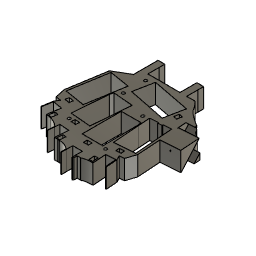
Copy_v4 (Autodesk Fusion 360 design; units mm, degrees)
Autodesk Fusion 360 part; units mm, degrees
note: some values were not read from the file. Set by a fixed rule: which sketch regions a step uses.
other "Base Mesh Feature1"
sketch "Sketch1" plane through (0, 0, 0.01) normal (0, 0, 1) x (1, 0, 0)
  line L0 (36.0813, -1.8889) -> (32.9752, 43.2487)
  line L1 (32.7513, -12.1179) -> (36.0813, -1.8889)
  line L2 (27.6845, -12.4899) -> (32.7513, -12.1179)
  line L3 (30.0654, -16.8996) -> (27.6845, -12.4899)
  line L4 (30.9849, -29.0009) -> (30.0654, -16.8996)
  line L5 (29.4427, -17.4772) -> (30.3023, -29.0109)
  line L6 (19.6436, -18.2077) -> (29.4427, -17.4772)
  line L7 (20.6901, -32.2445) -> (19.6436, -18.2077)
  line L8 (6.3028, -33.911) -> (9.753, -33.9098)
  line L9 (6.3027, -37.2346) -> (6.3028, -33.911)
  line L10 (5.577, -37.9174) -> (6.3027, -37.2346)
  line L11 (4.9263, -37.9059) -> (5.577, -37.9174)
  line L12 (4.9132, -27.2369) -> (4.9059, -37.8615)
  line L13 (-4.9131, -27.2369) -> (4.9132, -27.2369)
  line L14 (-4.9303, -38.8327) -> (-4.9131, -27.2369)
  line L15 (-5.5394, -38.808) -> (-4.9303, -38.8327)
  line L16 (-5.5099, -33.2116) -> (-5.5394, -38.808)
  line L17 (-18.1322, -29.3561) -> (-16.5345, -29.3675)
  line L18 (-21.6433, -29.2745) -> (-18.1322, -29.3561)
  line L19 (-20.4904, -15.7696) -> (-21.6433, -29.2745)
  line L20 (-30.2811, -14.9338) -> (-20.4904, -15.7696)
  line L21 (-31.2834, -26.4889) -> (-30.2811, -14.9338)
  line L22 (-31.7337, -26.4423) -> (-31.2834, -26.4889)
  line L23 (-31.1662, -19.694) -> (-31.7337, -26.4423)
  line L24 (-46.0317, -13.0034) -> (-45.6993, -13.1615)
  line L25 (-43.8507, 0.1867) -> (-46.0317, -13.0034)
  line L26 (-53.5454, 1.7898) -> (-43.8507, 0.1867)
  line L27 (-55.2865, -8.7399) -> (-53.5454, 1.7898)
  line L28 (-55.8526, -8.6917) -> (-55.2865, -8.7399)
  line L29 (-54.0371, 2.3883) -> (-55.8526, -8.6917)
  line L30 (-51.2811, 6.5583) -> (-54.0371, 2.3883)
  line L31 (-56.4897, 7.4399) -> (-51.2811, 6.5583)
  line L32 (-58.7948, 17.9104) -> (-56.4897, 7.4399)
  line L33 (-52.3403, 57.6045) -> (-58.7948, 17.9104)
  line L34 (-36.826, 66.678) -> (-52.3403, 57.6045)
  line L35 (-36.8289, 85.8904) -> (-36.826, 66.678)
  line L36 (-29.9469, 74.4662) -> (-29.9469, 85.8904)
  line L37 (2.7431, 74.4567) -> (-29.9469, 74.4662)
  line L38 (2.7431, 85.8904) -> (2.7431, 74.4567)
  line L39 (9.6191, 85.8904) -> (2.7431, 85.8904)
  line L40 (9.6191, 74.4567) -> (9.6191, 85.8904)
  line L41 (18.0806, 74.4608) -> (9.6191, 74.4567)
  line L42 (40.9354, 52.3159) -> (40.995, 53.4081)
  line L43 (43.4569, 50.4105) -> (40.9354, 52.3159)
  line L44 (44.0171, 50.8716) -> (43.4569, 50.4105)
  line L45 (42.0183, 41.437) -> (45.9172, 41.6472)
  line L46 (32.9752, 43.2487) -> (42.0183, 41.437)
  line L47 (20.5159, 63.3141) -> (16.3615, 42.6858)
  line L48 (-18.6487, 70.9533) -> (20.5159, 63.3141)
  line L49 (-22.6664, 50.5546) -> (-18.6487, 70.9533)
  line L50 (16.3615, 42.6858) -> (-22.6664, 50.5546)
  line L51 (4.9059, -37.8615) -> (4.9263, -37.9059)
  spline S0 degree 5 poles (45.9172, 41.6472) (46.0239, 42.1861) (46.222, 43.1941) (46.4734, 44.4972) (46.6984, 45.8908) (46.6354, 47.3689) (46.0898, 48.5946) (45.2491, 49.6596) (44.4651, 50.4535) (44.0171, 50.8716) knots 0 0 0 0 0 0 0.2 0.4 0.6 0.8 1 1 1 1 1 1
  line L52 (45.063, 49.8956) -> (42.9712, 51.8475)
  line L53 (45.6555, 40.3248) -> (46.179, 42.9695)
  line L54 (-29.9469, 85.8904) -> (-36.8289, 85.8904)
  line L55 (9.7581, -34.0874) -> (9.753, -33.9098)
  line L56 (30.9849, -29.0009) -> (30.3023, -29.0109)
  spline S1 degree 5 poles (40.995, 53.4081) (38.5459, 54.9422) (34.2281, 57.7327) (29.4904, 61.0866) (26.0623, 64.1864) (24.207, 66.9799) (22.775, 69.3323) (20.8665, 71.6268) (19.0929, 73.4647) (18.0806, 74.4608) knots 0 0 0 0 0 0 0.2 0.4 0.6 0.8 1 1 1 1 1 1
  line L57 (47.1881, 49.5288) -> (34.8019, 57.2874)
  line L58 (20.6612, 71.9215) -> (15.5, 77)
  spline S2 degree 5 poles (20.6901, -32.2445) (20.1069, -32.2354) (18.9879, -32.2293) (17.4506, -32.2564) (15.6408, -32.3648) (13.618, -32.6511) (12.0778, -33.0579) (10.9226, -33.5077) (10.1472, -33.8818) (9.7581, -34.0874) knots 0 0 0 0 0 0 0.2 0.4 0.6 0.8 1 1 1 1 1 1
  line L59 (10.7258, -33.576) -> (8.7904, -34.5988)
  line L60 (22.1647, -32.2674) -> (19.2154, -32.2215)
  line L61 (18.766, -24.9684) -> (19.1881, -30.9501)
  line L62 (15.1693, -25.251) -> (18.766, -24.9684)
  line L63 (15.5913, -31.2369) -> (15.1693, -25.251)
  line L64 (19.1881, -30.9501) -> (15.5913, -31.2369)
  line L65 (-2.4635, -18.739) -> (2.4519, -18.7391)
  line L66 (-2.4564, -14.9483) -> (-2.4635, -18.739)
  line L67 (2.4519, -14.9483) -> (-2.4564, -14.9483)
  line L68 (2.4519, -18.7391) -> (2.4519, -14.9483)
  line L69 (21.4548, -9.5512) -> (26.3566, -9.1859)
  line L70 (21.1801, -5.7705) -> (21.4548, -9.5512)
  line L71 (26.0748, -5.4057) -> (21.1801, -5.7705)
  line L72 (26.3566, -9.1859) -> (26.0748, -5.4057)
  line L73 (-16.2753, -22.8856) -> (-16.7887, -28.8562)
  line L74 (-19.6716, -22.5382) -> (-16.2753, -22.8856)
  line L75 (-20.1856, -28.5134) -> (-19.6716, -22.5382)
  line L76 (-16.7887, -28.8562) -> (-20.1856, -28.5134)
  line L77 (-21.8975, -3.3162) -> (-22.2199, -7.0932)
  line L78 (-26.7951, -2.8981) -> (-21.8975, -3.3162)
  line L79 (-27.1175, -6.6751) -> (-26.7951, -2.8981)
  line L80 (-22.2199, -7.0932) -> (-27.1175, -6.6751)
  spline S3 degree 5 poles (-5.5099, -33.2116) (-5.8497, -32.9739) (-6.5527, -32.5017) (-7.6769, -31.8034) (-9.3011, -30.9072) (-11.507, -29.9489) (-13.4115, -29.4433) (-14.9328, -29.2986) (-15.993, -29.3242) (-16.5345, -29.3675) knots 0 0 0 0 0 0 0.2 0.4 0.6 0.8 1 1 1 1 1 1
  line L81 (-4.6593, -33.8068) -> (-6.3605, -32.6165)
  line L82 (-15.2099, -29.2615) -> (-17.8592, -29.4735)
  spline S4 degree 5 poles (-31.1662, -19.694) (-31.3545, -19.3593) (-31.8362, -18.6888) (-32.8739, -17.6793) (-34.8089, -16.3455) (-37.895, -14.8239) (-40.7733, -13.8723) (-43.148, -13.4044) (-44.832, -13.2211) (-45.6993, -13.1615) knots 0 0 0 0 0 0 0.2 0.4 0.6 0.8 1 1 1 1 1 1
  line L83 (-43.5543, -13.3088) -> (-47.8443, -13.0143)
  line L84 (-30.7289, -20.4713) -> (-31.6035, -18.9166)
  line L85 (-40.0467, -7.1995) -> (-41.0386, -13.1166)
  line L86 (-43.5618, -6.6259) -> (-40.0467, -7.1995)
  line L87 (-44.5531, -12.5388) -> (-43.5618, -6.6259)
  line L88 (-41.0386, -13.1166) -> (-44.5531, -12.5388)
  circle A0 centre (-30.7678, -4.9879) radius 1.4659
  circle A1 centre (14.7861, -13.3473) radius 1.4659
  line L89 (-10.5247, -12.0229) -> (10.5003, -12.0259)
  line L90 (-10.5102, 27.8914) -> (-10.5247, -12.0229)
  line L91 (9.6517, 27.8914) -> (-10.5102, 27.8914)
  line L92 (10.1905, 24.0869) -> (9.6517, 27.8914)
  line L93 (10.5003, -12.0259) -> (10.1905, 24.0869)
  line L94 (22.4476, 37.2561) -> (30.9201, 37.9127)
  line L95 (30.9201, 37.9127) -> (33.9307, -1.9021)
  line L96 (33.9307, -1.9021) -> (12.9473, -3.4609)
  line L97 (12.9473, -3.4609) -> (9.9887, 36.3068)
  line L98 (9.9887, 36.3068) -> (18.4543, 36.9595)
  line L99 (18.4543, 36.9595) -> (18.5275, 35.9515)
  line L100 (18.5275, 35.9515) -> (22.5161, 36.2534)
  line L101 (22.5161, 36.2534) -> (22.4476, 37.2561)
  line L102 (-10.2152, 38.6652) -> (-13.611, -1.0998)
  line L103 (-30.4568, 40.4222) -> (-10.2152, 38.6652)
  line L104 (-31.4926, 36.7486) -> (-30.4568, 40.4222)
  line L105 (-34.5584, 0.7056) -> (-31.4926, 36.7486)
  line L106 (-13.611, -1.0998) -> (-34.5584, 0.7056)
  circle A2 centre (4.6568, 34.6748) radius 1.5
  line L107 (-44.8927, 8.9723) -> (-49.7422, 9.7741)
  line L108 (-49.7422, 9.7741) -> (-49.1168, 13.5129)
  line L109 (-49.1168, 13.5129) -> (-44.2743, 12.7122)
  line L110 (-44.2743, 12.7122) -> (-44.8927, 8.9723)
  line L111 (-35.8494, 14.2954) -> (-56.6063, 17.7506)
  line L112 (-56.6063, 17.7506) -> (-50.1165, 56.9742)
  line L113 (-50.1165, 56.9742) -> (-29.3405, 53.5561)
  line L114 (-29.3405, 53.5561) -> (-35.8494, 14.2954)
  line L115 (24.536, 49.2635) -> (20.8213, 50.0184)
  line L116 (20.8213, 50.0184) -> (21.7896, 54.8302)
  line L117 (21.7896, 54.8302) -> (25.5057, 54.0823)
  line L118 (25.5057, 54.0823) -> (24.536, 49.2635)
  circle A3 centre (-25.4932, 45.1036) radius 1.5
  circle A4 centre (-25.2593, 67.4913) radius 1.5
  constraint midpoint L44.start L52
  constraint midpoint L45.end L53
  constraint midpoint L42.end L57
  constraint midpoint L41.start L58
  constraint midpoint L55.start L59
  constraint midpoint L7.start L60
  constraint midpoint L16.start L81
  constraint midpoint L17.end L82
  constraint midpoint L24.end L83
  constraint midpoint L23.start L84
other "MeshSection1"
extrude "Extrude1" add sketch "Sketch1" along normal blind 19.73 makes body 1
extrude "Extrude2" add 1 faces at (7.3271, 85.8904, 6.5867) along direction (-0.000001, 1, 0) blind 5.8 on bodies 1 bodies 1
extrude "Extrude3" add 1 faces at (-34.5349, 85.8904, 13.1633) along direction (-0.000001, 1, 0) blind 5.8 on bodies 1 bodies 1
other "GenerateFaceGroups1"
sketch "Sketch1 (2)" plane through (0, 0, 0.01) normal (0, 0, -1) x (1, 0, 0) in component "pouce"
  line L0 (25.5057, -54.0823) -> (21.7896, -54.8302)
  line L1 (21.7896, -54.8302) -> (20.8213, -50.0184)
  line L2 (20.8213, -50.0184) -> (24.536, -49.2635)
  line L3 (24.536, -49.2635) -> (25.5057, -54.0823)
  line L4 (10.5003, 12.0259) -> (10.1905, -24.0869)
  line L5 (10.1905, -24.0869) -> (9.6517, -27.8914)
  line L6 (9.6517, -27.8914) -> (-10.5102, -27.8914)
  line L7 (-10.5102, -27.8914) -> (-10.5247, 12.0229)
  line L8 (-10.5247, 12.0229) -> (10.5003, 12.0259)
  line L9 (-41.0386, 13.1166) -> (-40.0467, 7.1995)
  line L10 (-40.0467, 7.1995) -> (-43.5618, 6.6259)
  line L11 (-43.5618, 6.6259) -> (-44.5531, 12.5388)
  line L12 (-44.5531, 12.5388) -> (-41.0386, 13.1166)
  circle A0 centre (-25.2593, -67.4913) radius 1.5
  line L13 (2.4519, 18.7391) -> (2.4519, 14.9483)
  line L14 (2.4519, 14.9483) -> (-2.4564, 14.9483)
  line L15 (-2.4564, 14.9483) -> (-2.4635, 18.739)
  line L16 (-2.4635, 18.739) -> (2.4519, 18.7391)
  line L17 (-13.611, 1.0998) -> (-10.2152, -38.6652)
  line L18 (-10.2152, -38.6652) -> (-30.4568, -40.4222)
  line L19 (-30.4568, -40.4222) -> (-31.4926, -36.7486)
  line L20 (-31.4926, -36.7486) -> (-34.5584, -0.7056)
  line L21 (-34.5584, -0.7056) -> (-13.611, 1.0998)
  circle A1 centre (14.7861, 13.3473) radius 1.4659
  line L22 (-44.2743, -12.7122) -> (-49.1168, -13.5129)
  line L23 (-49.1168, -13.5129) -> (-49.7422, -9.7741)
  line L24 (-49.7422, -9.7741) -> (-44.8927, -8.9723)
  line L25 (-44.8927, -8.9723) -> (-44.2743, -12.7122)
  circle A2 centre (-30.7678, 4.9879) radius 1.4659
  line L26 (22.5161, -36.2534) -> (18.5275, -35.9515)
  line L27 (18.5275, -35.9515) -> (18.4543, -36.9595)
  line L28 (18.4543, -36.9595) -> (9.9887, -36.3068)
  line L29 (9.9887, -36.3068) -> (12.9473, 3.4609)
  line L30 (12.9473, 3.4609) -> (33.9307, 1.9021)
  line L31 (33.9307, 1.9021) -> (30.9201, -37.9127)
  line L32 (30.9201, -37.9127) -> (22.4476, -37.2561)
  line L33 (22.4476, -37.2561) -> (22.5161, -36.2534)
  circle A3 centre (4.6568, -34.6748) radius 1.5
  circle A4 centre (-25.4932, -45.1036) radius 1.5
  line L34 (-29.3405, -53.5561) -> (-50.1165, -56.9742)
  line L35 (-50.1165, -56.9742) -> (-56.6063, -17.7506)
  line L36 (-56.6063, -17.7506) -> (-35.8494, -14.2954)
  line L37 (-35.8494, -14.2954) -> (-29.3405, -53.5561)
  line L38 (19.1881, 30.9501) -> (18.766, 24.9684)
  line L39 (18.766, 24.9684) -> (15.1693, 25.251)
  line L40 (15.1693, 25.251) -> (15.5913, 31.2369)
  line L41 (15.5913, 31.2369) -> (19.1881, 30.9501)
  line L42 (26.3566, 9.1859) -> (26.0748, 5.4057)
  line L43 (26.0748, 5.4057) -> (21.1801, 5.7705)
  line L44 (21.1801, 5.7705) -> (21.4548, 9.5512)
  line L45 (21.4548, 9.5512) -> (26.3566, 9.1859)
  line L46 (16.3615, -42.6858) -> (20.5159, -63.3141)
  line L47 (20.5159, -63.3141) -> (-18.6487, -70.9533)
  line L48 (-18.6487, -70.9533) -> (-22.6664, -50.5546)
  line L49 (-22.6664, -50.5546) -> (16.3615, -42.6858)
  line L50 (-16.7887, 28.8562) -> (-16.2753, 22.8856)
  line L51 (-16.2753, 22.8856) -> (-19.6716, 22.5382)
  line L52 (-19.6716, 22.5382) -> (-20.1856, 28.5134)
  line L53 (-20.1856, 28.5134) -> (-16.7887, 28.8562)
  line L54 (-22.2199, 7.0932) -> (-21.8975, 3.3162)
  line L55 (-21.8975, 3.3162) -> (-26.7951, 2.8981)
  line L56 (-26.7951, 2.8981) -> (-27.1175, 6.6751)
  line L57 (-27.1175, 6.6751) -> (-22.2199, 7.0932)
  line L58 (-31.2834, 26.4889) -> (-31.7337, 26.4423)
  line L59 (-31.7337, 26.4423) -> (-31.1662, 19.694)
  spline S0 degree 5 poles (-31.1662, 19.694) (-31.3545, 19.3593) (-31.8362, 18.6888) (-32.8739, 17.6793) (-34.8089, 16.3455) (-37.895, 14.8239) (-40.7733, 13.8723) (-43.148, 13.4044) (-44.832, 13.2211) (-45.6993, 13.1615) knots 0 0 0 0 0 0 0.2 0.4 0.6 0.8 1 1 1 1 1 1
  line L60 (-45.6993, 13.1615) -> (-46.0317, 13.0034)
  line L61 (-46.0317, 13.0034) -> (-43.8507, -0.1867)
  line L62 (-43.8507, -0.1867) -> (-53.5454, -1.7898)
  line L63 (-53.5454, -1.7898) -> (-55.2865, 8.7399)
  line L64 (-55.2865, 8.7399) -> (-55.8526, 8.6917)
  line L65 (-55.8526, 8.6917) -> (-54.0371, -2.3883)
  line L66 (-54.0371, -2.3883) -> (-51.2811, -6.5583)
  line L67 (-51.2811, -6.5583) -> (-56.4897, -7.4399)
  line L68 (-56.4897, -7.4399) -> (-58.7948, -17.9104)
  line L69 (-58.7948, -17.9104) -> (-52.3403, -57.6045)
  line L70 (-52.3403, -57.6045) -> (-36.826, -66.678)
  line L71 (-36.826, -66.678) -> (-36.8289, -85.8904)
  line L72 (-36.8289, -85.8904) -> (-36.8289, -91.6904)
  line L73 (-36.8289, -91.6904) -> (-29.9469, -91.6904)
  line L74 (-29.9469, -91.6904) -> (-29.9469, -85.8904)
  line L75 (-29.9469, -85.8904) -> (-29.9469, -74.4662)
  line L76 (-29.9469, -74.4662) -> (2.7431, -74.4567)
  line L77 (2.7431, -74.4567) -> (2.7431, -85.8904)
  line L78 (2.7431, -85.8904) -> (2.7431, -91.6904)
  line L79 (2.7431, -91.6904) -> (9.6191, -91.6904)
  line L80 (9.6191, -91.6904) -> (9.6191, -85.8904)
  line L81 (9.6191, -85.8904) -> (9.6191, -74.4567)
  line L82 (9.6191, -74.4567) -> (18.0806, -74.4608)
  spline S1 degree 5 poles (40.995, -53.4081) (38.5459, -54.9422) (34.2281, -57.7327) (29.4904, -61.0866) (26.0623, -64.1864) (24.207, -66.9799) (22.775, -69.3323) (20.8665, -71.6268) (19.0929, -73.4647) (18.0806, -74.4608) knots 0 0 0 0 0 0 0.2 0.4 0.6 0.8 1 1 1 1 1 1
  line L83 (40.995, -53.4081) -> (40.9354, -52.3159)
  line L84 (40.9354, -52.3159) -> (43.4569, -50.4105)
  line L85 (43.4569, -50.4105) -> (44.0171, -50.8716)
  spline S2 degree 5 poles (45.9172, -41.6472) (46.0239, -42.1861) (46.222, -43.1941) (46.4734, -44.4972) (46.6984, -45.8908) (46.6354, -47.3689) (46.0898, -48.5946) (45.2491, -49.6596) (44.4651, -50.4535) (44.0171, -50.8716) knots 0 0 0 0 0 0 0.2 0.4 0.6 0.8 1 1 1 1 1 1
  line L86 (45.9172, -41.6472) -> (42.0183, -41.437)
  line L87 (42.0183, -41.437) -> (32.9752, -43.2487)
  line L88 (32.9752, -43.2487) -> (36.0813, 1.8889)
  line L89 (36.0813, 1.8889) -> (32.7513, 12.1179)
  line L90 (32.7513, 12.1179) -> (27.6845, 12.4899)
  line L91 (27.6845, 12.4899) -> (30.0654, 16.8996)
  line L92 (30.0654, 16.8996) -> (30.9849, 29.0009)
  line L93 (30.9849, 29.0009) -> (30.3023, 29.0109)
  line L94 (30.3023, 29.0109) -> (29.4427, 17.4772)
  line L95 (29.4427, 17.4772) -> (19.6436, 18.2077)
  line L96 (19.6436, 18.2077) -> (20.6901, 32.2445)
  spline S3 degree 5 poles (20.6901, 32.2445) (20.1069, 32.2354) (18.9879, 32.2293) (17.4506, 32.2564) (15.6408, 32.3648) (13.618, 32.6511) (12.0778, 33.0579) (10.9226, 33.5077) (10.1472, 33.8818) (9.7581, 34.0874) knots 0 0 0 0 0 0 0.2 0.4 0.6 0.8 1 1 1 1 1 1
  line L97 (9.7581, 34.0874) -> (9.753, 33.9098)
  line L98 (9.753, 33.9098) -> (6.3028, 33.911)
  line L99 (6.3028, 33.911) -> (6.3027, 37.2346)
  line L100 (6.3027, 37.2346) -> (5.577, 37.9174)
  line L101 (5.577, 37.9174) -> (4.9263, 37.9059)
  line L102 (4.9263, 37.9059) -> (4.9059, 37.8615)
  line L103 (4.9059, 37.8615) -> (4.9132, 27.2369)
  line L104 (4.9132, 27.2369) -> (-4.9131, 27.2369)
  line L105 (-4.9131, 27.2369) -> (-4.9303, 38.8327)
  line L106 (-4.9303, 38.8327) -> (-5.5394, 38.808)
  line L107 (-5.5394, 38.808) -> (-5.5099, 33.2116)
  spline S4 degree 5 poles (-5.5099, 33.2116) (-5.8497, 32.9739) (-6.5527, 32.5017) (-7.6769, 31.8034) (-9.3011, 30.9072) (-11.507, 29.9489) (-13.4115, 29.4433) (-14.9328, 29.2986) (-15.993, 29.3242) (-16.5345, 29.3675) knots 0 0 0 0 0 0 0.2 0.4 0.6 0.8 1 1 1 1 1 1
  line L108 (-16.5345, 29.3675) -> (-18.1322, 29.3561)
  line L109 (-18.1322, 29.3561) -> (-21.6433, 29.2745)
  line L110 (-21.6433, 29.2745) -> (-20.4904, 15.7696)
  line L111 (-20.4904, 15.7696) -> (-30.2811, 14.9338)
  line L112 (-30.2811, 14.9338) -> (-31.2834, 26.4889)
  line L113 (20.5159, -63.3141) -> (29.2219, -61.5608)
  line L114 (37.4968, -42.3428) -> (17.119, -46.4467)
  constraint coincident L46.end L47.start
  constraint coincident S1 L113.end
  constraint perpendicular L46 L113
  constraint midpoint L87 L114.start
  constraint coincident L46 L114.end
  constraint perpendicular L46 L114
extrude "Extrude1'" add sketch "Sketch1 (2)" along normal blind 10 separate body contours L46 S1 L83 L84 L85 S2 L86 L87 L113 L114 makes body 2 in component "pouce"
extrude "Extrude2'" add 1 faces at (18.2513, 52.0692, -6.6567) along direction (-0.980318, 0.197427, 0) blind 15 on bodies 2 bodies 2 in component "pouce"
copy_body "Body->Comp1" bodies 1 removing the originals makes body 3 in component "Hand"
sketch "Sketch2" plane through (35.7818, 2.4622, 0) normal (0.997641, 0.06865, 0) x (-0.06865, 0.997641, 0) in component "pouce"
  line L0 (-4.3614, 0.01) -> (40.8829, 0.01)
  line L1 (40.8829, 0.01) -> (40.8829, 19.74)
  line L2 (40.8829, 19.74) -> (-4.3614, 19.74)
  line L3 (-4.3614, 19.74) -> (-4.3614, 0.01)
  line L4 (47.749, 0.01) -> (10.0415, 0.01)
  line L5 (10.0415, 0.01) -> (10.0415, 19.74)
  line L6 (10.0415, 19.74) -> (47.749, 19.74)
  line L7 (47.749, 19.74) -> (47.749, 0.01)
  constraint horizontal L4
  constraint vertical L5
  constraint horizontal L6
  constraint vertical L7
  constraint coincident L2 L5.end
sketch "Sketch1 (3)" plane through (35.7818, 2.4622, 0) normal (0.997641, 0.06865, 0) x (-0.06865, 0.997641, 0) in component "Hand"
  line L0 (-4.3614, 0.01) -> (40.8829, 0.01)
  line L1 (40.8829, 0.01) -> (40.8829, 19.74)
  line L2 (40.8829, 19.74) -> (-4.3614, 19.74)
  line L3 (-4.3614, 19.74) -> (-4.3614, 0.01)
  line L4 (40.8829, 0.01) -> (19.8777, 0.01)
  line L5 (19.8777, 0.01) -> (19.8777, 19.74)
  line L6 (19.8777, 19.74) -> (40.8829, 19.74)
  line L7 (40.8829, 19.74) -> (40.8829, 0.01)
  constraint horizontal L4
  constraint vertical L5
  constraint horizontal L6
  constraint vertical L7
  constraint coincident L2 L5.end
  constraint coincident L0.end L1.start
extrude "Extrude1''" add sketch "Sketch1 (3)" along normal blind 20 contours L0 L1 L2 L4 L5 L6 L7 bodies 3 in component "Hand"
sketch "Sketch2 (2)" plane through (55.7347, 3.8352, 0) normal (0.997641, 0.06865, 0) x (-0.06865, 0.997641, 0) in component "Hand"
  line L0 (40.8829, 19.74) -> (19.8777, 19.74)
  line L1 (19.8777, 19.74) -> (19.8777, 0.01)
  line L2 (19.8777, 0.01) -> (40.8829, 0.01)
  line L3 (40.8829, 0.01) -> (40.8829, 19.74)
  line L4 (40.8829, 6.3559) -> (34.537, 0.01)
  line L5 (40.8829, 6.3559) -> (49.8574, 6.3559) construction
  line L6 (40.8829, 6.3559) -> (51.3779, 16.8509)
  line L7 (24.537, 25.01) -> (34.537, 25.01)
  line L8 (51.3779, 16.8509) -> (44.3068, 23.922)
  line L9 (51.3779, 16.8509) -> (61.3779, 16.8509) construction
  line L10 (44.3068, 23.922) -> (20.3948, 0.01)
  dimension "d15" = 135
  dimension "d17" = 25
  dimension "d18" = 135
  dimension "d19" = 10
  dimension "d20" = 90
  constraint horizontal L5
  constraint coincident L3 L4.start
  constraint coincident L2 L4.end
  constraint parallel L4 L6
  constraint horizontal L7
  constraint horizontal L9
  constraint coincident L2 L10.end
  measures "d15" angle of L4 L5
  measures "d17" distance of L4.end L7.end
  measures "d18" angle of L8 L9
  measures "d19" distance of L6.end L8.end
  measures "d20" angle of L8 L10
extrude "Extrude2''" cut sketch "Sketch2 (2)" against normal blind 20 contours L0 L2 L3 L4 L10 | L0 L3 L6 L8 L10 bodies 3 in component "Hand"
sketch "Sketch3" plane through (-0.6997, 10.1684, -10.1924) normal (-0.048543, 0.705439, -0.707107) x (-0.997641, -0.06865, 0) in component "Hand"
  line L0 (-35.8665, 42.3308) -> (-55.8665, 42.3308)
  line L1 (-55.8665, 42.3308) -> (-55.8665, 14.4284)
  line L2 (-55.8665, 14.4284) -> (-35.8665, 14.4284)
  line L3 (-35.8665, 14.4284) -> (-35.8665, 42.3308)
  line L4 (-35.8665, 14.4284) -> (-55.8665, 34.4284)
  line L5 (-35.8665, 14.4284) -> (-7.5822, 14.4284) construction
  circle A0 centre (-45.8665, 24.4284) radius 0.5
  dimension "d23" = 135
  dimension "d24" = 1
  constraint horizontal L5
  constraint coincident L2.end L3.start
  constraint coincident L1 L4.end
  constraint midpoint L4 A0.centre
  measures "d23" angle of L4 L5
  measures "d24" diameter of A0
extrude "Extrude3'" cut sketch "Sketch3" along normal blind 56.5 and the other way blind 19 contours L4 A0 | L4 A0 bodies 3 in component "Hand"
component "pouce" placed x (1, 0, 0) y (0, 1, 0) z (0, 0, 1) at (0, 0, 0)
component "Hand" placed x (1, 0, 0) y (0, 1, 0) z (0, 0, 1) at (0, 0, 0)
